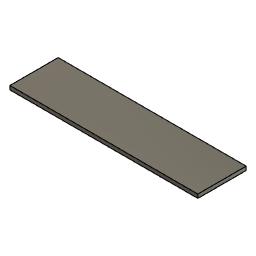
Tissue mount flat 10mm v2 (Autodesk Fusion 360 design; units mm, degrees)
Autodesk Fusion 360 part; units mm, degrees
sketch "Sketch1" plane through (0, 0, 0) normal (0, 1, 0) x (1, 0, 0)
  line L0 (0, 0) -> (35, 0)
  line L1 (35, 0) -> (35, -9)
  line L2 (35, -9) -> (0, -9)
  line L3 (0, -9) -> (0, 0)
  dimension "d1" = 35
  dimension "d2" = 9
  constraint horizontal L0
  constraint vertical L1
  constraint horizontal L2
  constraint vertical L3
  constraint coincident L0.start L3.end
  measures "d1" distance of L0.start L0.end
  measures "d2" distance of L0.start L2.end
extrude "Extrude1" add sketch "Sketch1" along normal blind 0.5
extrude "Extrude2" add 1 faces at (11.6667, 0.5, 3) along direction (0, 1, 0) blind 0.2
